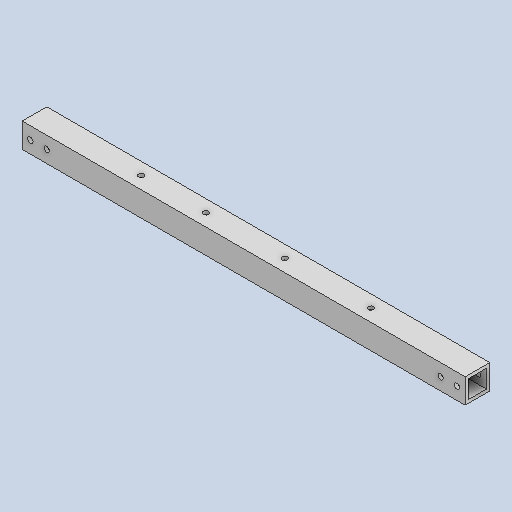
# Autodesk Inventor part: light_kaku_2020
Saved by Autodesk Inventor 2025.2 (Build 292293000, 293)
## iProperties
Created: 2025-05-05
Part Number: light_kaku_2020
Material: 一般
Document SubType Name: Modeling
Designer: yuki0520
Density: 1 g/cm^3
Appearance: 既定
Author: yuki0520
Autodesk Inventor part; units mm, degrees
ref_plane "YZ Plane" through (0, 0, 0) normal (1, 0, 0) x (0, 1, 0)
ref_plane "XZ Plane" through (0, 0, 0) normal (0, 1, 0) x (-1, 0, 0)
ref_plane "XY Plane" through (0, 0, 0) normal (0, 0, 1) x (1, 0, 0)
derived "zzz_light_plate.ipt"
sketch "スケッチ1" plane through (0, 0, 0) normal (0, 0, 1) x (1, 0, 0)
  circle A0 centre (0, 0) radius 120
  line L0 (12.25, 120) -> (-12.25, 120)
  line L1 (-12.25, 120) -> (-12.25, 196)
  line L2 (-12.25, 196) -> (12.25, 196)
  line L3 (12.25, 196) -> (12.25, 120)
  line L4 (12.25, 120) -> (-12.25, 196) construction
  line L5 (-12.25, 120) -> (12.25, 196) construction
  line L6 (-41.25, 158) -> (95.75, 158)
  line L7 (0, -120) -> (0, 120)
  line L8 (59.75, 218) -> (59.75, 138)
  circle A1 centre (400, 0) radius 120
  circle A2 centre (400, 158) radius 38
  line L9 (400, -120) -> (400, 120)
  line L10 (-120, 0) -> (120, 0)
  circle A3 centre (400, 158) radius 16
  circle A4 centre (400, 190) radius 16
  circle A5 centre (400, 190) radius 12
  line L11 (102.75, 178) -> (59.75, 178)
  line L12 (59.75, 178) -> (59.75, 202)
  line L13 (59.75, 202) -> (102.75, 202)
  line L14 (102.75, 202) -> (102.75, 178)
  line L15 (102.75, 178) -> (59.75, 202) construction
  line L16 (59.75, 178) -> (102.75, 202) construction
  line L17 (57.75, 218) -> (57.75, 121.8661)
  circle A6 centre (400, 190) radius 9.5
  circle A7 centre (400, 190) radius 6.55
  circle A8 centre (404.3332, 198.4542) radius 1.3
  circle A9 centre (390.5119, 189.5255) radius 1.3
  circle A10 centre (405.155, 182.0203) radius 1.3
  line L18 (135, 218) -> (-135, 218)
  line L19 (-135, 218) -> (-135, 203)
  line L20 (-135, 203) -> (135, 203)
  line L21 (135, 203) -> (135, 218)
  circle A11 centre (400, 158) radius 7.5
  line L22 (-35.25, 218) -> (-35.25, 138)
  line L23 (22.25, 218) -> (22.25, 138)
  line L24 (17.25, 138) -> (17.25, 218)
  line L25 (-30.25, 218) -> (-30.25, 138)
  line L26 (12.25, -196) -> (12.25, -120)
  line L27 (12.25, -120) -> (-12.25, -196) construction
  line L28 (-12.25, -120) -> (-12.25, -196)
  line L29 (12.25, -120) -> (-12.25, -120)
  line L30 (-12.25, -120) -> (12.25, -196) construction
  line L31 (-12.25, -196) -> (12.25, -196)
  line L32 (17.25, -138) -> (17.25, -218)
  line L33 (-41.25, -158) -> (95.75, -158)
  line L34 (-135, -203) -> (135, -203)
  line L35 (135, -218) -> (-135, -218)
  line L36 (57.75, -218) -> (57.75, -121.8661)
  line L37 (135, -203) -> (135, -218)
  line L38 (59.75, -218) -> (59.75, -138)
  line L39 (22.25, -218) -> (22.25, -138)
  line L40 (59.75, -178) -> (59.75, -202)
  line L41 (102.75, -178) -> (59.75, -178)
  line L42 (102.75, -178) -> (59.75, -202) construction
  line L43 (102.75, -202) -> (102.75, -178)
  line L44 (59.75, -178) -> (102.75, -202) construction
  line L45 (-35.25, -218) -> (-35.25, -138)
  line L46 (-135, -218) -> (-135, -203)
  line L47 (-30.25, -218) -> (-30.25, -138)
  line L48 (46.75, -182) -> (56.75, -182)
  line L49 (60, -182) -> (50, -182)
  line L50 (59.75, -202) -> (102.75, -202)
  line L51 (46.75, -134) -> (56.75, -182) construction
  line L52 (56.75, -134) -> (46.75, -134)
  line L53 (56.75, -182) -> (56.75, -134)
  line L54 (46.75, -134) -> (46.75, -182)
  line L55 (56.75, -134) -> (46.75, -182) construction
  line L56 (-135, 203) -> (-135, -203)
  line L57 (453, 189) -> (438, 189)
  line L58 (438, 189) -> (438, 174)
  line L59 (438, 174) -> (453, 174)
  line L60 (453, 174) -> (453, 189)
  line L61 (438, 158) -> (438, -0.316)
  circle A12 centre (480, 0) radius 120
  line L62 (605, 50) -> (600, 50)
  line L63 (600, 50) -> (600, -50)
  line L64 (600, -50) -> (605, -50)
  line L65 (605, -50) -> (605, 50)
  line L66 (438, 174) -> (453, 174)
  line L67 (453, 174) -> (453, 169)
  line L68 (453, 169) -> (438, 169)
  line L69 (438, 169) -> (438, 174)
  arc A13 (600, 50) -> (453, 169) centre (359.7884, -96.4378) ccw
  line L70 (438, 189) -> (453, 189)
  line L71 (453, 189) -> (453, 194)
  line L72 (453, 194) -> (438, 194)
  line L73 (438, 194) -> (438, 189)
  arc A14 (605, 50) -> (453, 194) centre (369.2063, -46.6712) ccw
  circle A15 centre (400, 136.2498) radius 38
  circle A16 centre (420, 190) radius 3
  circle A17 centre (400, 190) radius 20
  circle A18 centre (400, 210) radius 3
  circle A19 centre (380, 190) radius 3
  line L74 (438, 169) -> (410.2848, 145.7434)
  line L75 (438, 194) -> (401.3623, 212.6729)
  line L76 (397.8787, 212.1213) -> (377.8787, 192.1213)
  line L77 (384.3412, 154.7133) -> (377.064, 189.3837)
  line L78 (57.75, 193) -> (40.75, 193)
  line L79 (40.75, 193) -> (40.75, 187)
  line L80 (40.75, 187) -> (57.75, 187)
  line L81 (57.75, 187) -> (57.75, 193)
  line L82 (102.75, 190) -> (81.25, 190)
  line L83 (22.25, 167) -> (23.25, 167)
  line L84 (23.25, 167) -> (23.25, 149)
  line L85 (23.25, 149) -> (22.25, 149)
  line L86 (22.25, 149) -> (22.25, 167)
  line L87 (23.25, 166.5) -> (30.75, 166.5)
  line L88 (30.75, 166.5) -> (30.75, 149.5)
  line L89 (30.75, 149.5) -> (23.25, 149.5)
  line L90 (23.25, 149.5) -> (23.25, 166.5)
  line L91 (37.75, 174) -> (42.75, 174)
  line L92 (42.75, 174) -> (42.75, 142)
  line L93 (42.75, 142) -> (37.75, 142)
  line L94 (37.75, 142) -> (37.75, 174)
  line L95 (37.75, 174) -> (42.75, 174)
  line L96 (42.75, 174) -> (42.75, 206)
  line L97 (42.75, 206) -> (37.75, 206)
  line L98 (37.75, 206) -> (37.75, 174)
  line L99 (37.75, 190) -> (42.75, 190)
  line L100 (42.75, 200) -> (52.75, 200)
  line L101 (52.75, 200) -> (52.75, 180)
  line L102 (52.75, 180) -> (42.75, 180)
  line L103 (42.75, 180) -> (42.75, 200)
  point P0 (0, 158)
  point P1 (0, -158)
  point P2 (51.75, -158)
  point P3 (65.8106, -158)
extrude "押し出し1" add sketch "スケッチ1" along normal blind 15 contours L24 L18 L23 L20 | L20 L25 L18 L24 | L20 L22 L18 L25 | L23 L18 L17 L20 L96 L97 L98 | L20 L19 L18 L22 | L98 L97 L96 L20 | L18 L8 L20 L17 | L18 L21 L20 L8
sketch "スケッチ2" plane through (-135, 218, 0) normal (0, 1, 0) x (1, 0, 0)
  line L0 (270, 0) -> (0, 0) projected
  line L1 (0, 0) -> (270, 0) projected
  line L2 (270, 0) -> (0, 0) projected
  line L3 (0, 0) -> (0, -15) projected
  line L4 (270, -15) -> (0, -15) projected
  line L5 (270, 0) -> (270, -15) projected
  line L6 (0, -7.5) -> (270, -7.5)
  point P0 (135, 0)
  point P1 (205, -7.5)
  point P2 (152.5, -7.5)
  point P3 (104.5, -7.5)
  point P4 (99.75, 0)
  point P5 (99.75, 0)
  point P6 (99.75, 0)
  point P7 (157.25, 0)
  point P8 (157.25, 0)
  point P9 (157.25, 0)
  point P10 (152.25, 0)
  point P11 (152.25, 0)
  point P12 (152.25, 0)
  point P13 (104.75, 0)
  point P14 (104.75, 0)
  point P15 (104.75, 0)
  point P16 (65, -7.5)
  point P17 (135, -7.5)
  dimension "d31" = 140
  dimension "d32" = 70
  dimension "d33" = 17.5
  dimension "d34" = 30.5
  constraints: 4 point on line, 3 midpoint, 2 end point, 1 other
  measures "d31" distance of point (65, -7.5) point (205, -7.5)
  measures "d32" distance of point (135, -7.5) point (205, -7.5)
  measures "d33" distance of point (135, -7.5) point (152.5, -7.5)
  measures "d34" distance of point (104.5, -7.5) point (135, -7.5)
hole "穴1" at (-30.5, 218, 7.5) at (17.5, 218, 7.5) at (70, 218, 7.5) at (-70, 218, 7.5) direction (0, -1, 0) diameter 3.3 end through all
sketch "スケッチ3" plane through (135, 203, 0) normal (1, 0, 0) x (0, 0, -1)
  line L0 (0, 0) -> (0, 15) projected
  line L1 (0, 15) -> (-15, 15) projected
  line L2 (-15, 0) -> (-15, 15) projected
  line L3 (0, 0) -> (-15, 0) projected
  line L4 (-13, 13) -> (-2, 13)
  line L5 (-2, 13) -> (-2, 2)
  line L6 (-2, 2) -> (-13, 2)
  line L7 (-13, 2) -> (-13, 13)
  point P0 (0, -203)
  dimension "d15" = 2
  constraints: 8 end point, 3 other
  measures "d15" distance between parallel lines of L1 L4
extrude "押し出し2" cut sketch "スケッチ3" against normal blind 400 contours L4 L5 L6 L7
sketch "スケッチ4" plane through (-135, 218, 15) normal (0, 0, 1) x (1, 0, 0)
  line L0 (270, 0) -> (0, 0) projected
  line L1 (0, 0) -> (0, -15) projected
  line L2 (0, -15) -> (270, -15) projected
  line L3 (270, -15) -> (270, 0) projected
  line L4 (0, -7.5) -> (270, -7.5)
  point P0 (135, -218)
  point P1 (5, -7.5)
  point P2 (15, -7.5)
  point P3 (265, -7.5)
  point P4 (255, -7.5)
  dimension "d18" = 10
  dimension "d19" = 5
  dimension "d20" = 10
  dimension "d21" = 5
  constraints: 4 point on line, 2 end point, 2 midpoint
  measures "d18" distance of point (265, -7.5) point (255, -7.5)
  measures "d19" distance from line of L3 point (265, -7.5)
  measures "d20" distance of point (5, -7.5) point (15, -7.5)
  measures "d21" distance from line of L1 point (5, -7.5)
hole "穴2" at (-130, 210.5, 15) at (-120, 210.5, 15) at (130, 210.5, 15) at (120, 210.5, 15) direction (0, 0, -1) diameter 3.3 end through all
equation "\"d32\" = 0.5 * d31"
